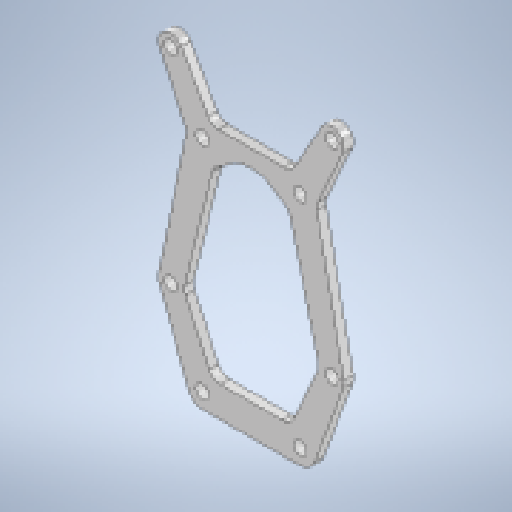
# Autodesk Inventor part: matasita
Saved by Autodesk Inventor 2025.1 (Build 291241000, 241)
## iProperties
Created: 2024-09-02
Part Number: matasita
Material: アルミニウム 2014-T4
Document SubType Name: Modeling
Designer: right
Density: 2.8 g/cm^3
Appearance: サテン
Mass: 2.30251 g
Surface Area: 15.601 cm^2
Volume: 0.822325 cm^3
Author: right
Autodesk Inventor part; units mm, degrees
ref_plane "YZ Plane" through (0, 0, 0) normal (1, 0, 0) x (0, 1, 0)
ref_plane "XZ Plane" through (0, 0, 0) normal (0, 1, 0) x (-1, 0, 0)
ref_plane "XY Plane" through (0, 0, 0) normal (0, 0, 1) x (1, 0, 0)
sketch "スケッチ1" plane through (0, 0, 0) normal (0, 0, 1) x (1, 0, 0)
  circle A0 centre (4, -6) radius 1.05
  circle A1 centre (4, -6) radius 1.1
  circle A2 centre (20, -6) radius 1.05
  circle A3 centre (20, -42) radius 1.1
  circle A4 centre (4, -42) radius 1.05
  circle A5 centre (20, -6) radius 1.1
  circle A6 centre (20, -42) radius 1.1
  circle A7 centre (4, -42) radius 1.1
  circle A8 centre (4, -42) radius 2.5
  circle A9 centre (20, -42) radius 2.5
  circle A10 centre (20, -6) radius 2.5
  circle A11 centre (4, -6) radius 2.5
  arc A12 (-0.741742, -29.885509) -> (-0.741742, -28.614491) centre (-1.2, -29.25) ccw
  arc A13 (24.741742, -28.614491) -> (24.741742, -29.885509) centre (25.2, -29.25) ccw
  arc A14 (-0.741742, 3.614491) -> (-0.741742, 4.885509) centre (-1.2, 4.25) ccw
  arc A15 (24.741742, 4.885509) -> (24.741742, 3.614491) centre (25.2, 4.25) ccw
  line L0 (24.741742, 5.75) -> (24.741742, 4.885509)
  line L1 (24.741742, 5.75) -> (22.7, 5.75)
  line L2 (22.7, 5.75) -> (22.7, 2.75)
  line L3 (24.741742, 2.75) -> (22.7, 2.75)
  line L4 (24.741742, 3.614491) -> (24.741742, 2.75)
  circle A16 centre (-1.2, 4.25) radius 1.1
  circle A17 centre (25.2, 4.25) radius 1.1
  circle A18 centre (25.2, -29.25) radius 1.1
  circle A19 centre (-1.2, -29.25) radius 1.1
  circle A20 centre (-1.2, -29.25) radius 2
  circle A21 centre (25.2, -29.25) radius 2
  circle A22 centre (25.2, 4.25) radius 2
  circle A23 centre (-1.2, 4.25) radius 2
  line L5 (-3.078107, -29.937542) -> (1.652366, -42.859427)
  line L6 (0.623256, -28.427966) -> (6.279069, -40.972458)
  line L7 (4, -39.5) -> (20, -39.5)
  line L8 (20, -44.5) -> (4, -44.5)
  line L9 (0.742189, -29.727393) -> (6.427736, -6.596741)
  line L10 (-3.160511, -28.854531) -> (1.549361, -5.505664)
  line L11 (-3.021278, 3.423595) -> (1.723402, -7.033006)
  line L12 (6.17819, -4.773016) -> (0.542552, 5.231587)
  line L13 (4, -3.5) -> (20, -3.5)
  line L14 (20, -8.5) -> (4, -8.5)
  line L15 (17.82181, -4.773016) -> (23.457448, 5.231587)
  line L16 (27.021278, 3.423595) -> (22.276598, -7.033006)
  line L17 (17.572264, -6.596741) -> (23.257811, -29.727393)
  line L18 (27.160511, -28.854531) -> (22.450639, -5.505664)
  line L19 (23.376744, -28.427966) -> (17.720931, -40.972458)
  line L20 (27.078107, -29.937542) -> (22.347634, -42.859427)
  circle A24 centre (12, -12.5) radius 6.232545
  point P0 (0, 0)
  point P1 (5.615196, -39.5)
  point P2 (0.906933, -29.057158)
  point P3 (5.959912, -8.5)
  point P4 (18.040088, -8.5)
  point P5 (23.093067, -29.057158)
  point P6 (18.384804, -39.5)
  point P7 (18.538906, -3.5)
  point P8 (5.461094, -3.5)
  point P9 (1.389644, -6.29745)
  point P10 (22.610356, -6.29745)
  point P11 (7.220396, -8.5)
  point P12 (16.779604, -8.5)
  dimension "d0" = 2.2
  dimension "d1" = 2.2
  dimension "d2" = 2.2
  dimension "d3" = 2.2
  dimension "d4" = 5
  dimension "d5" = 5
  dimension "d6" = 5
  dimension "d7" = 5
  dimension "d8" = 2.2
  dimension "d9" = 2.2
  dimension "d10" = 2.2
  dimension "d11" = 2.2
  dimension "d12" = 4
  dimension "d13" = 4
  dimension "d14" = 4
  dimension "d15" = 4
  constraints: 32 end point, 32 point on circle, 32 tangent, 16 centre point, 16 coincident
  measures "d0" diameter of A1
  measures "d1" diameter of A5
  measures "d2" diameter of A6
  measures "d3" diameter of A7
  measures "d4" diameter of A8
  measures "d5" diameter of A9
  measures "d6" diameter of A10
  measures "d7" diameter of A11
  measures "d8" diameter of A16
  measures "d9" diameter of A17
  measures "d10" diameter of A18
  measures "d11" diameter of A19
  measures "d12" diameter of A20
  measures "d13" diameter of A21
  measures "d14" diameter of A22
  measures "d15" diameter of A23
sketch "スケッチ1 outline for 押し出し1" plane through (0, 0, 0) normal (0, 0, 1) x (1, 0, 0)
  arc A0 (27.021278, 3.423595) -> (23.457448, 5.231587) centre (25.2, 4.25) ccw
  line L0 (22.610356, -6.29745) -> (27.021278, 3.423595)
  line L1 (23.457448, 5.231587) -> (18.538906, -3.5)
  line L2 (27.160511, -28.854531) -> (22.610356, -6.29745)
  line L3 (18.538906, -3.5) -> (5.461094, -3.5)
  arc A1 (27.078107, -29.937542) -> (27.160511, -28.854531) centre (25.2, -29.25) ccw
  line L4 (5.461094, -3.5) -> (0.542552, 5.231587)
  line L5 (22.347634, -42.859427) -> (27.078107, -29.937542)
  arc A2 (0.542552, 5.231587) -> (-3.021278, 3.423595) centre (-1.2, 4.25) ccw
  arc A3 (20, -44.5) -> (22.347634, -42.859427) centre (20, -42) ccw
  line L6 (-3.021278, 3.423595) -> (1.389644, -6.29745)
  line L7 (4, -44.5) -> (20, -44.5)
  line L8 (1.389644, -6.29745) -> (-3.160511, -28.854531)
  arc A4 (1.652366, -42.859427) -> (4, -44.5) centre (4, -42) ccw
  arc A5 (-3.160511, -28.854531) -> (-3.078107, -29.937542) centre (-1.2, -29.25) ccw
  line L9 (-3.078107, -29.937542) -> (1.652366, -42.859427)
  circle A6 centre (4, -42) radius 1.1
  circle A7 centre (-1.2, -29.25) radius 1.1
  circle A8 centre (20, -42) radius 1.1
  line L10 (5.615196, -39.5) -> (0.906933, -29.057158)
  line L11 (18.384804, -39.5) -> (5.615196, -39.5)
  line L12 (23.093067, -29.057158) -> (18.384804, -39.5)
  line L13 (18.040088, -8.5) -> (23.093067, -29.057158)
  line L14 (16.779604, -8.5) -> (18.040088, -8.5)
  arc A9 (7.220396, -8.5) -> (16.779604, -8.5) centre (12, -12.5) cw
  line L15 (5.959912, -8.5) -> (7.220396, -8.5)
  line L16 (0.906933, -29.057158) -> (5.959912, -8.5)
  circle A10 centre (25.2, -29.25) radius 1.1
  circle A11 centre (4, -6) radius 1.1
  circle A12 centre (-1.2, 4.25) radius 1.1
  circle A13 centre (20, -6) radius 1.1
  circle A14 centre (25.2, 4.25) radius 1.1
extrude "押し出し1" add sketch "スケッチ1 outline for 押し出し1" along normal blind 1.5
fillet "フィレット1" radius 2 12 edges at (0.9069, -29.0572, 0.75) (5.6152, -39.5, 0.75) (18.3848, -39.5, 0.75) (23.0931, -29.0572, 0.75) (18.0401, -8.5, 0.75) (5.9599, -8.5, 0.75) (7.2204, -8.5, 0.75) (16.7796, -8.5, 0.75) (5.4611, -3.5, 0.75) (18.5389, -3.5, 0.75) (1.3896, -6.2975, 0.75) (22.6104, -6.2975, 0.75)
